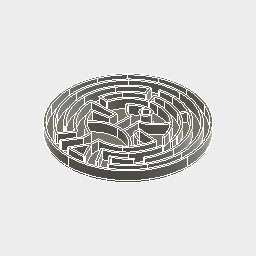
Maze (Autodesk Fusion 360 design; units mm, degrees)
Autodesk Fusion 360 part; units mm, degrees
sketch "Sketch5" plane through (0, 0, 0) normal (0, 1, 0) x (1, 0, 0)
  spline S0 degree 3 poles (-3.4402, 73.5513) (-20.4265, 73.5513) (-36.3809, 66.9367) (-48.3929, 54.9246) knots 0 0 0 0 1 1 1 1
  spline S1 degree 3 poles (-48.3929, 54.9246) (-60.405, 42.9125) (-66.9932, 26.9846) (-66.9932, 9.9983) knots 0 0 0 0 1 1 1 1
  spline S2 degree 3 poles (-66.9932, 9.9983) (-66.9932, -1.3523) (-63.9504, -12.4912) (-58.2354, -22.2279) knots 0 0 0 0 1 1 1 1
  spline S3 degree 3 poles (-58.2354, -22.2279) (-52.6792, -31.6735) (-44.7152, -39.5581) (-35.2167, -45.0615) knots 0 0 0 0 1 1 1 1
  spline S4 degree 3 poles (-35.2167, -45.0615) (-34.7404, -45.326) (-34.1319, -45.1937) (-33.8144, -44.7439) knots 0 0 0 0 1 1 1 1
  line L0 (-33.8144, -44.7439) -> (-23.9984, -30.8269)
  spline S5 degree 3 poles (-23.9984, -30.8269) (-23.6544, -30.3506) (-23.7867, -29.6892) (-24.2629, -29.3452) knots 0 0 0 0 1 1 1 1
  spline S6 degree 3 poles (-24.2629, -29.3452) (-24.2894, -29.3188) (-24.3423, -29.3188) (-24.3688, -29.2923) knots 0 0 0 0 1 1 1 1
  spline S7 degree 3 poles (-24.3688, -29.2923) (-37.8096, -21.8575) (-46.5673, -6.9085) (-46.8848, 8.9665) knots 0 0 0 0 1 1 1 1
  line L1 (-46.8848, 8.9665) -> (-20.9027, 9.9454)
  line L2 (-20.9027, 9.9454) -> (-20.9027, 4.786)
  line L3 (-20.9027, 4.786) -> (-38.1271, 1.7963)
  spline S8 degree 3 poles (-38.1271, 1.7963) (-38.7356, 1.6904) (-39.1325, 1.0554) (-38.9738, 0.4733) knots 0 0 0 0 1 1 1 1
  spline S9 degree 3 poles (-38.9738, 0.4733) (-35.8782, -11.1154) (-27.3586, -20.4023) (-16.1402, -24.5298) knots 0 0 0 0 1 1 1 1
  line L4 (-16.1402, -24.5298) -> (-16.1402, -32.8377)
  line L5 (-16.1402, -32.8377) -> (-25.7711, -48.1835)
  spline S10 degree 3 poles (-25.7711, -48.1835) (-26.0886, -48.6863) (-25.9298, -49.3213) (-25.4271, -49.6388) knots 0 0 0 0 1 1 1 1
  spline S11 degree 3 poles (-25.4271, -49.6388) (-25.2419, -49.7446) (-25.0567, -49.7975) (-24.8715, -49.7975) knots 0 0 0 0 1 1 1 1
  spline S12 degree 3 poles (-24.8715, -49.7975) (-24.5275, -49.7975) (-24.1836, -49.6123) (-23.9719, -49.2948) knots 0 0 0 0 1 1 1 1
  line L6 (-23.9719, -49.2948) -> (-14.0236, -33.4198)
  line L7 (-14.0236, -33.4198) -> (-14.0236, -23.7625)
  spline S13 degree 3 poles (-14.0236, -23.7625) (-14.0236, -23.3127) (-14.3146, -22.9158) (-14.738, -22.7571) knots 0 0 0 0 1 1 1 1
  spline S14 degree 3 poles (-14.738, -22.7571) (-19.7915, -21.0108) (-24.263, -18.1798) (-27.9407, -14.5285) knots 0 0 0 0 1 1 1 1
  spline S15 degree 3 poles (-27.9407, -14.5285) (-22.0934, -6.935) (-12.9917, -2.4106) (-3.4403, -2.4106) knots 0 0 0 0 1 1 1 1
  spline S16 degree 3 poles (-3.4403, -2.4106) (6.8785, -2.4106) (15.5568, -6.6704) (21.1131, -14.4756) knots 0 0 0 0 1 1 1 1
  spline S17 degree 3 poles (21.1131, -14.4756) (20.0018, -15.825) (18.8377, -16.9627) (17.6735, -17.8888) knots 0 0 0 0 1 1 1 1
  spline S18 degree 3 poles (17.6735, -17.8888) (12.0379, -22.3867) (4.9471, -24.6621) (-3.4402, -24.6621) knots 0 0 0 0 1 1 1 1
  spline S19 degree 3 poles (-3.4402, -24.6621) (-4.0223, -24.6621) (-4.4986, -25.1383) (-4.4986, -25.7204) knots 0 0 0 0 1 1 1 1
  line L8 (-4.4986, -25.7204) -> (-4.4986, -34.4517)
  line L9 (-4.4986, -34.4517) -> (-13.6267, -51.0675)
  spline S20 degree 3 poles (-13.6267, -51.0675) (-13.8119, -51.385) (-13.8119, -51.7819) (-13.6002, -52.1258) knots 0 0 0 0 1 1 1 1
  spline S21 degree 3 poles (-13.6002, -52.1258) (-13.415, -52.4433) (-13.0711, -52.655) (-12.7006, -52.655) knots 0 0 0 0 1 1 1 1
  line L10 (-12.7006, -52.655) -> (5.291, -52.655)
  spline S22 degree 3 poles (5.291, -52.655) (5.6614, -52.655) (6.0054, -52.4698) (6.1906, -52.1523) knots 0 0 0 0 1 1 1 1
  spline S23 degree 3 poles (6.1906, -52.1523) (6.3758, -51.8348) (6.4023, -51.4379) (6.2171, -51.1204) knots 0 0 0 0 1 1 1 1
  line L11 (6.2171, -51.1204) -> (-2.3819, -34.4517)
  line L12 (-2.3819, -34.4517) -> (-2.3819, -26.7523)
  spline S24 degree 3 poles (-2.3819, -26.7523) (6.0318, -26.5671) (13.2021, -24.1594) (18.9964, -19.5556) knots 0 0 0 0 1 1 1 1
  spline S25 degree 3 poles (18.9964, -19.5556) (25.0289, -14.7667) (30.6381, -4.5008) (33.3104, 6.5852) knots 0 0 0 0 1 1 1 1
  spline S26 degree 3 poles (33.3104, 6.5852) (33.3898, 6.8762) (33.3104, 7.1937) (33.1516, 7.4319) knots 0 0 0 0 1 1 1 1
  spline S27 degree 3 poles (33.1516, 7.4319) (32.9664, 7.67) (32.7018, 7.8552) (32.4108, 7.8817) knots 0 0 0 0 1 1 1 1
  line L13 (32.4108, 7.8817) -> (10.9796, 10.2629)
  spline S28 degree 3 poles (10.9796, 10.2629) (10.6885, 10.2894) (10.371, 10.21) (10.1594, 9.9983) knots 0 0 0 0 1 1 1 1
  spline S29 degree 3 poles (10.1594, 9.9983) (9.9477, 9.7867) (9.8154, 9.5221) (9.8154, 9.2046) knots 0 0 0 0 1 1 1 1
  line L14 (9.8154, 9.2046) -> (9.8154, 2.8546)
  spline S30 degree 3 poles (9.8154, 2.8546) (9.8154, 2.4577) (10.0535, 2.0608) (10.4239, 1.9021) knots 0 0 0 0 1 1 1 1
  line L15 (10.4239, 1.9021) -> (20.531, -2.8604)
  spline S31 degree 3 poles (20.531, -2.8604) (21.0602, -3.0985) (21.6952, -2.8869) (21.9333, -2.3577) knots 0 0 0 0 1 1 1 1
  spline S32 degree 3 poles (21.9333, -2.3577) (22.1714, -1.8285) (21.9598, -1.1935) (21.4306, -0.9554) knots 0 0 0 0 1 1 1 1
  line L16 (21.4306, -0.9554) -> (11.9056, 3.516)
  line L17 (11.9056, 3.516) -> (11.9056, 8.014)
  line L18 (11.9056, 8.014) -> (30.9556, 5.8973)
  spline S33 degree 3 poles (30.9556, 5.8973) (29.1035, -1.2465) (26.0079, -7.914) (22.4625, -12.7558) knots 0 0 0 0 1 1 1 1
  spline S34 degree 3 poles (22.4625, -12.7558) (17.7529, -6.4323) (11.0854, -2.3577) (3.1744, -0.9025) knots 0 0 0 0 1 1 1 1
  line L19 (3.1744, -0.9025) -> (3.1744, 16.269)
  spline S35 degree 3 poles (3.1744, 16.269) (11.6146, 18.174) (18.4937, 26.6671) (23.1504, 33.4669) knots 0 0 0 0 1 1 1 1
  spline S36 degree 3 poles (23.1504, 33.4669) (25.6639, 30.6887) (27.6748, 27.4873) (29.0506, 23.9154) knots 0 0 0 0 1 1 1 1
  spline S37 degree 3 poles (29.0506, 23.9154) (30.4529, 20.3171) (30.4529, 20.3171) (31.1937, 16.5071) knots 0 0 0 0 1 1 1 1
  line L20 (31.1937, 16.5071) -> (31.2202, 16.4012)
  spline S38 degree 3 poles (31.2202, 16.4012) (31.326, 15.8985) (31.7493, 15.5546) (32.2521, 15.5546) knots 0 0 0 0 1 1 1 1
  spline S39 degree 3 poles (32.2521, 15.5546) (32.3314, 15.5546) (32.3843, 15.5546) (32.4637, 15.581) knots 0 0 0 0 1 1 1 1
  spline S40 degree 3 poles (32.4637, 15.581) (33.0458, 15.6869) (33.4162, 16.2425) (33.2839, 16.8246) knots 0 0 0 0 1 1 1 1
  line L21 (33.2839, 16.8246) -> (33.2575, 16.9304)
  spline S41 degree 3 poles (33.2575, 16.9304) (32.4637, 20.8727) (32.4373, 20.9521) (31.0085, 24.6827) knots 0 0 0 0 1 1 1 1
  spline S42 degree 3 poles (31.0085, 24.6827) (25.8227, 38.0971) (12.3025, 46.7754) (-3.4402, 46.7754) knots 0 0 0 0 1 1 1 1
  spline S43 degree 3 poles (-3.4402, 46.7754) (-6.3771, 46.7754) (-9.2346, 46.4315) (-11.9863, 45.77) knots 0 0 0 0 1 1 1 1
  line L22 (-11.9863, 45.77) -> (-13.7854, 52.1729)
  spline S44 degree 3 poles (-13.7854, 52.1729) (-10.3723, 53.0196) (-6.8533, 53.4429) (-3.3079, 53.4429) knots 0 0 0 0 1 1 1 1
  spline S45 degree 3 poles (-3.3079, 53.4429) (3.386, 53.4429) (9.7889, 52.0406) (15.7156, 49.3154) knots 0 0 0 0 1 1 1 1
  spline S46 degree 3 poles (15.7156, 49.3154) (26.2725, 44.4206) (34.1306, 35.8217) (37.8877, 25.0531) knots 0 0 0 0 1 1 1 1
  spline S47 degree 3 poles (37.8877, 25.0531) (38.311, 23.836) (38.6021, 23.0423) (38.8137, 22.4602) knots 0 0 0 0 1 1 1 1
  spline S48 degree 3 poles (38.8137, 22.4602) (39.3958, 20.8992) (39.4752, 20.714) (40.2425, 16.9304) knots 0 0 0 0 1 1 1 1
  spline S49 degree 3 poles (40.2425, 16.9304) (40.3483, 16.4277) (40.7717, 16.0838) (41.2744, 16.0838) knots 0 0 0 0 1 1 1 1
  spline S50 degree 3 poles (41.2744, 16.0838) (41.3537, 16.0838) (41.4067, 16.0838) (41.486, 16.1102) knots 0 0 0 0 1 1 1 1
  spline S51 degree 3 poles (41.486, 16.1102) (42.0681, 16.2161) (42.4385, 16.7717) (42.3062, 17.3538) knots 0 0 0 0 1 1 1 1
  spline S52 degree 3 poles (42.3062, 17.3538) (41.5125, 21.2961) (41.4066, 21.5871) (40.7981, 23.2275) knots 0 0 0 0 1 1 1 1
  spline S53 degree 3 poles (40.7981, 23.2275) (40.56, 23.8361) (40.2954, 24.5769) (39.8721, 25.7675) knots 0 0 0 0 1 1 1 1
  spline S54 degree 3 poles (39.8721, 25.7675) (36.2208, 36.2979) (28.786, 44.8704) (18.8377, 50.1621) knots 0 0 0 0 1 1 1 1
  line L23 (18.8377, 50.1621) -> (21.6423, 56.1681)
  spline S55 degree 3 poles (21.6423, 56.1681) (38.6021, 46.9342) (49.0796, 29.3659) (49.0796, 10.0248) knots 0 0 0 0 1 1 1 1
  spline S56 degree 3 poles (49.0796, 10.0248) (49.0796, 0.7115) (46.6189, -8.4166) (41.9358, -16.4071) knots 0 0 0 0 1 1 1 1
  spline S57 degree 3 poles (41.9358, -16.4071) (41.6448, -16.9098) (41.8035, -17.5712) (42.3062, -17.8623) knots 0 0 0 0 1 1 1 1
  spline S58 degree 3 poles (42.3062, -17.8623) (42.465, -17.9681) (42.6502, -17.9946) (42.8354, -17.9946) knots 0 0 0 0 1 1 1 1
  spline S59 degree 3 poles (42.8354, -17.9946) (43.2058, -17.9946) (43.5498, -17.8094) (43.7614, -17.4654) knots 0 0 0 0 1 1 1 1
  spline S60 degree 3 poles (43.7614, -17.4654) (48.6033, -9.1575) (51.1698, 0.3675) (51.1698, 10.0513) knots 0 0 0 0 1 1 1 1
  spline S61 degree 3 poles (51.1698, 10.0513) (51.1698, 30.5565) (39.8456, 49.1567) (21.6158, 58.6023) knots 0 0 0 0 1 1 1 1
  spline S62 degree 3 poles (21.6158, 58.6023) (13.9164, 62.5975) (5.2381, 64.6877) (-3.4667, 64.6877) knots 0 0 0 0 1 1 1 1
  spline S63 degree 3 poles (-3.4667, 64.6877) (-8.2556, 64.6877) (-13.0181, 64.0527) (-17.6219, 62.8356) knots 0 0 0 0 1 1 1 1
  spline S64 degree 3 poles (-17.6219, 62.8356) (-18.1775, 62.6769) (-18.5215, 62.0948) (-18.3627, 61.5392) knots 0 0 0 0 1 1 1 1
  spline S65 degree 3 poles (-18.3627, 61.5392) (-18.204, 60.9836) (-17.6219, 60.6396) (-17.0663, 60.7984) knots 0 0 0 0 1 1 1 1
  spline S66 degree 3 poles (-17.0663, 60.7984) (-12.6477, 61.989) (-8.0704, 62.5711) (-3.4667, 62.5711) knots 0 0 0 0 1 1 1 1
  spline S67 degree 3 poles (-3.4667, 62.5711) (4.6825, 62.5711) (12.4877, 60.7454) (19.7373, 57.1736) knots 0 0 0 0 1 1 1 1
  line L24 (19.7373, 57.1736) -> (16.9327, 51.0881)
  spline S68 degree 3 poles (16.9327, 51.0881) (16.8268, 51.141) (16.721, 51.194) (16.5887, 51.2469) knots 0 0 0 0 1 1 1 1
  spline S69 degree 3 poles (16.5887, 51.2469) (10.3975, 54.1308) (3.6771, 55.586) (-3.3344, 55.586) knots 0 0 0 0 1 1 1 1
  spline S70 degree 3 poles (-3.3344, 55.586) (-7.4354, 55.586) (-11.4836, 55.0569) (-15.3994, 53.9721) knots 0 0 0 0 1 1 1 1
  spline S71 degree 3 poles (-15.3994, 53.9721) (-15.955, 53.8133) (-16.299, 53.2312) (-16.1402, 52.6756) knots 0 0 0 0 1 1 1 1
  spline S72 degree 3 poles (-16.1402, 52.6756) (-16.1402, 52.6492) (-16.1402, 52.6492) (-16.1138, 52.6227) knots 0 0 0 0 1 1 1 1
  spline S73 degree 3 poles (-16.1138, 52.6227) (-16.1138, 52.5962) (-16.1138, 52.5962) (-16.1138, 52.5698) knots 0 0 0 0 1 1 1 1
  line L25 (-16.1138, 52.5698) -> (-14.05, 45.2144)
  spline S74 degree 3 poles (-14.05, 45.2144) (-25.7446, 41.6954) (-35.2167, 32.4614) (-38.7621, 20.3435) knots 0 0 0 0 1 1 1 1
  line L26 (-38.7621, 20.3435) -> (-45.5619, 20.714)
  spline S75 degree 3 poles (-45.5619, 20.714) (-44.0538, 26.6406) (-41.2492, 32.2762) (-37.4127, 37.0652) knots 0 0 0 0 1 1 1 1
  spline S76 degree 3 poles (-37.4127, 37.0652) (-33.3646, 42.1187) (-28.1523, 46.2992) (-22.3315, 49.1302) knots 0 0 0 0 1 1 1 1
  spline S77 degree 3 poles (-22.3315, 49.1302) (-21.8288, 49.3683) (-21.5906, 49.9504) (-21.8023, 50.4531) knots 0 0 0 0 1 1 1 1
  line L27 (-21.8023, 50.4531) -> (-25.1096, 58.9463)
  spline S78 degree 3 poles (-25.1096, 58.9463) (-25.2155, 59.2108) (-25.4271, 59.4225) (-25.6917, 59.5548) knots 0 0 0 0 1 1 1 1
  spline S79 degree 3 poles (-25.6917, 59.5548) (-25.9563, 59.6606) (-26.2738, 59.6606) (-26.5384, 59.5283) knots 0 0 0 0 1 1 1 1
  spline S80 degree 3 poles (-26.5384, 59.5283) (-35.8252, 55.1892) (-43.6834, 48.3365) (-49.2925, 39.711) knots 0 0 0 0 1 1 1 1
  spline S81 degree 3 poles (-49.2925, 39.711) (-55.034, 30.874) (-58.0767, 20.5817) (-58.0767, 9.9983) knots 0 0 0 0 1 1 1 1
  spline S82 degree 3 poles (-58.0767, 9.9983) (-58.0767, -6.1942) (-50.9594, -21.4342) (-38.5505, -31.8588) knots 0 0 0 0 1 1 1 1
  spline S83 degree 3 poles (-38.5505, -31.8588) (-38.3652, -32.0175) (-38.1007, -32.0969) (-37.8625, -32.0969) knots 0 0 0 0 1 1 1 1
  spline S84 degree 3 poles (-37.8625, -32.0969) (-37.5715, -32.0969) (-37.254, -31.9646) (-37.0423, -31.7265) knots 0 0 0 0 1 1 1 1
  spline S85 degree 3 poles (-37.0423, -31.7265) (-36.6719, -31.2767) (-36.7248, -30.6152) (-37.1746, -30.2448) knots 0 0 0 0 1 1 1 1
  spline S86 degree 3 poles (-37.1746, -30.2448) (-49.1073, -20.2171) (-55.9336, -5.5592) (-55.9336, 9.9983) knots 0 0 0 0 1 1 1 1
  spline S87 degree 3 poles (-55.9336, 9.9983) (-55.9336, 20.1848) (-53.0232, 30.0537) (-47.4934, 38.5733) knots 0 0 0 0 1 1 1 1
  spline S88 degree 3 poles (-47.4934, 38.5733) (-42.3075, 46.5373) (-35.1109, 52.9402) (-26.6442, 57.1206) knots 0 0 0 0 1 1 1 1
  line L28 (-26.6442, 57.1206) -> (-24.0777, 50.5854)
  spline S89 degree 3 poles (-24.0777, 50.5854) (-29.8192, 47.6485) (-34.9786, 43.4417) (-39.0002, 38.3881) knots 0 0 0 0 1 1 1 1
  spline S90 degree 3 poles (-39.0002, 38.3881) (-43.2865, 33.0171) (-46.3557, 26.6406) (-47.8638, 19.9467) knots 0 0 0 0 1 1 1 1
  spline S91 degree 3 poles (-47.8638, 19.9467) (-47.8638, 19.8937) (-47.8902, 19.8408) (-47.8902, 19.7614) knots 0 0 0 0 1 1 1 1
  spline S92 degree 3 poles (-47.8902, 19.7614) (-47.9167, 19.1794) (-47.4669, 18.6767) (-46.8848, 18.6502) knots 0 0 0 0 1 1 1 1
  line L29 (-46.8848, 18.6502) -> (-37.9684, 18.1739)
  spline S93 degree 3 poles (-37.9684, 18.1739) (-37.598, 18.1475) (-37.254, 18.3327) (-37.0423, 18.6502) knots 0 0 0 0 1 1 1 1
  spline S94 degree 3 poles (-37.0423, 18.6502) (-36.963, 18.756) (-36.91, 18.8619) (-36.8836, 18.9942) knots 0 0 0 0 1 1 1 1
  spline S95 degree 3 poles (-36.8836, 18.9942) (-33.6821, 30.9798) (-24.3688, 40.0814) (-12.833, 43.3358) knots 0 0 0 0 1 1 1 1
  spline S96 degree 3 poles (-12.833, 43.3358) (-12.78, 43.3358) (-12.7271, 43.3094) (-12.6742, 43.3094) knots 0 0 0 0 1 1 1 1
  spline S97 degree 3 poles (-12.6742, 43.3094) (-12.5684, 43.3094) (-12.489, 43.3094) (-12.3832, 43.3623) knots 0 0 0 0 1 1 1 1
  spline S98 degree 3 poles (-12.3832, 43.3623) (-12.2244, 43.4152) (-12.1186, 43.4681) (-11.9863, 43.5739) knots 0 0 0 0 1 1 1 1
  spline S99 degree 3 poles (-11.9863, 43.5739) (-9.2346, 44.2883) (-6.3507, 44.6587) (-3.3873, 44.6587) knots 0 0 0 0 1 1 1 1
  spline S100 degree 3 poles (-3.3873, 44.6587) (6.4552, 44.6587) (15.3716, 41.0869) (21.6952, 35.0014) knots 0 0 0 0 1 1 1 1
  spline S101 degree 3 poles (21.6952, 35.0014) (17.0914, 28.2281) (10.1858, 19.5498) (1.9837, 18.1739) knots 0 0 0 0 1 1 1 1
  spline S102 degree 3 poles (1.9837, 18.1739) (1.481, 18.0946) (1.1106, 17.6448) (1.1106, 17.1421) knots 0 0 0 0 1 1 1 1
  line L30 (1.1106, 17.1421) -> (1.1106, -0.585)
  spline S103 degree 3 poles (1.1106, -0.585) (-0.3446, -0.3998) (-1.8528, -0.3204) (-3.3873, -0.3204) knots 0 0 0 0 1 1 1 1
  spline S104 degree 3 poles (-3.3873, -0.3204) (-4.8161, -0.3204) (-6.2184, -0.4263) (-7.6207, -0.6115) knots 0 0 0 0 1 1 1 1
  line L31 (-7.6207, -0.6115) -> (-7.6207, 17.0892)
  spline S105 degree 3 poles (-7.6207, 17.0892) (-7.5942, 17.5919) (-7.9382, 18.0681) (-8.4409, 18.1739) knots 0 0 0 0 1 1 1 1
  spline S106 degree 3 poles (-8.4409, 18.1739) (-13.6796, 19.3117) (-17.913, 22.5396) (-21.379, 28.0165) knots 0 0 0 0 1 1 1 1
  spline S107 degree 3 poles (-21.379, 28.0165) (-17.8071, 31.5619) (-13.3886, 33.9431) (-8.5467, 34.9221) knots 0 0 0 0 1 1 1 1
  spline S108 degree 3 poles (-8.5467, 34.9221) (-9.2875, 33.8902) (-9.7373, 32.6467) (-9.7373, 31.2708) knots 0 0 0 0 1 1 1 1
  spline S109 degree 3 poles (-9.7373, 31.2708) (-9.7373, 27.8312) (-6.9592, 25.0531) (-3.5196, 25.0531) knots 0 0 0 0 1 1 1 1
  spline S110 degree 3 poles (-3.5196, 25.0531) (-0.0801, 25.0531) (2.6981, 27.8312) (2.6981, 31.2708) knots 0 0 0 0 1 1 1 1
  spline S111 degree 3 poles (2.6981, 31.2708) (2.6981, 34.6575) (-0.0271, 37.4092) (-3.3873, 37.4885) knots 0 0 0 0 1 1 1 1
  line L32 (-3.3873, 37.4885) -> (-3.3873, 37.5679)
  spline S112 degree 3 poles (-3.3873, 37.5679) (-11.0338, 37.5679) (-18.1511, 34.4987) (-23.4163, 28.969) knots 0 0 0 0 1 1 1 1
  spline S113 degree 3 poles (-23.4163, 28.969) (-23.4428, 28.9425) (-23.4428, 28.9425) (-23.4692, 28.916) knots 0 0 0 0 1 1 1 1
  spline S114 degree 3 poles (-23.4692, 28.916) (-23.7867, 28.5721) (-23.8661, 28.0694) (-23.6015, 27.646) knots 0 0 0 0 1 1 1 1
  spline S115 degree 3 poles (-23.6015, 27.646) (-19.9238, 21.5342) (-15.373, 17.83) (-9.7109, 16.3483) knots 0 0 0 0 1 1 1 1
  line L33 (-9.7109, 16.3483) -> (-9.7109, -0.9554)
  spline S116 degree 3 poles (-9.7109, -0.9554) (-17.3838, -2.49) (-24.3953, -6.7233) (-29.3165, -12.994) knots 0 0 0 0 1 1 1 1
  spline S117 degree 3 poles (-29.3165, -12.994) (-32.5709, -9.3162) (-35.058, -4.9242) (-36.5132, -0.0823) knots 0 0 0 0 1 1 1 1
  line L34 (-36.5132, -0.0823) -> (-18.6803, 3.0398)
  line L35 (-18.6803, 3.0398) -> (-18.6803, 12.1679)
  line L36 (-18.6803, 12.1679) -> (-47.9432, 11.0567)
  spline S118 degree 3 poles (-47.9432, 11.0567) (-48.5252, 11.0302) (-48.975, 10.554) (-48.9486, 9.9719) knots 0 0 0 0 1 1 1 1
  spline S119 degree 3 poles (-48.9486, 9.9719) (-48.9486, 9.9454) (-48.9486, 9.919) (-48.9486, 9.8925) knots 0 0 0 0 1 1 1 1
  line L37 (-48.9486, 9.8925) -> (-49.0279, 9.8925)
  spline S120 degree 3 poles (-49.0279, 9.8925) (-49.0279, -6.6704) (-40.1909, -22.4131) (-26.4061, -30.5358) knots 0 0 0 0 1 1 1 1
  line L38 (-26.4061, -30.5358) -> (-35.005, -42.7067)
  spline S121 degree 3 poles (-35.005, -42.7067) (-43.8156, -37.415) (-51.1975, -29.9802) (-56.4098, -21.1167) knots 0 0 0 0 1 1 1 1
  spline S122 degree 3 poles (-56.4098, -21.1167) (-61.9396, -11.724) (-64.8765, -0.929) (-64.8765, 10.0513) knots 0 0 0 0 1 1 1 1
  spline S123 degree 3 poles (-64.8765, 10.0513) (-64.8765, 26.4554) (-58.4736, 41.9071) (-46.8848, 53.4958) knots 0 0 0 0 1 1 1 1
  spline S124 degree 3 poles (-46.8848, 53.4958) (-35.2961, 65.0846) (-19.8444, 71.4875) (-3.4402, 71.4875) knots 0 0 0 0 1 1 1 1
  spline S125 degree 3 poles (-3.4402, 71.4875) (12.9639, 71.4875) (28.4156, 65.0846) (40.0044, 53.4958) knots 0 0 0 0 1 1 1 1
  spline S126 degree 3 poles (40.0044, 53.4958) (51.5931, 41.9071) (57.996, 26.4554) (57.996, 10.0513) knots 0 0 0 0 1 1 1 1
  spline S127 degree 3 poles (57.996, 10.0513) (57.996, -0.929) (55.0592, -11.6975) (49.5294, -21.1167) knots 0 0 0 0 1 1 1 1
  spline S128 degree 3 poles (49.5294, -21.1167) (44.2906, -30.0067) (36.8823, -37.4415) (28.0452, -42.7331) knots 0 0 0 0 1 1 1 1
  line L39 (28.0452, -42.7331) -> (22.78, -36.5419)
  spline S129 degree 3 poles (22.78, -36.5419) (28.0981, -33.4727) (34.5539, -29.6627) (38.3904, -25.0854) knots 0 0 0 0 1 1 1 1
  spline S130 degree 3 poles (38.3904, -25.0854) (38.7608, -24.6356) (38.7079, -23.9742) (38.2581, -23.6037) knots 0 0 0 0 1 1 1 1
  spline S131 degree 3 poles (38.2581, -23.6037) (37.8083, -23.2333) (37.1468, -23.2862) (36.7764, -23.736) knots 0 0 0 0 1 1 1 1
  spline S132 degree 3 poles (36.7764, -23.736) (33.0458, -28.181) (26.4841, -31.9646) (21.2454, -35.0073) knots 0 0 0 0 1 1 1 1
  line L40 (21.2454, -35.0073) -> (20.6369, -35.3512)
  spline S133 degree 3 poles (20.6369, -35.3512) (20.3723, -35.51) (20.1871, -35.7746) (20.1341, -36.0921) knots 0 0 0 0 1 1 1 1
  spline S134 degree 3 poles (20.1341, -36.0921) (20.0812, -36.4096) (20.1606, -36.7271) (20.3723, -36.9652) knots 0 0 0 0 1 1 1 1
  line L41 (20.3723, -36.9652) -> (27.0133, -44.7969)
  spline S135 degree 3 poles (27.0133, -44.7969) (27.225, -45.035) (27.516, -45.1673) (27.8335, -45.1673) knots 0 0 0 0 1 1 1 1
  spline S136 degree 3 poles (27.8335, -45.1673) (28.0187, -45.1673) (28.2039, -45.1144) (28.3627, -45.035) knots 0 0 0 0 1 1 1 1
  spline S137 degree 3 poles (28.3627, -45.035) (37.8612, -39.5581) (45.7987, -31.6471) (51.3814, -22.2014) knots 0 0 0 0 1 1 1 1
  spline S138 degree 3 poles (51.3814, -22.2014) (57.1229, -12.4648) (60.1391, -1.3258) (60.1391, 10.0248) knots 0 0 0 0 1 1 1 1
  spline S139 degree 3 poles (60.1391, 10.0248) (60.1391, 27.0111) (53.5245, 42.9654) (41.5125, 54.9775) knots 0 0 0 0 1 1 1 1
  spline S140 degree 3 poles (41.5125, 54.9775) (29.5004, 66.9631) (13.546, 73.5513) (-3.4402, 73.5513) knots 0 0 0 0 1 1 1 1
  line L42 (-10.9279, -50.5119) -> (-3.4667, -36.9652)
  line L43 (-3.4667, -36.9652) -> (3.5712, -50.5119)
  line L44 (3.5712, -50.5119) -> (-10.9279, -50.5119)
  spline S141 degree 3 poles (0.5285, 31.2973) (0.5285, 29.0483) (-1.3236, 27.1963) (-3.5725, 27.1963) knots 0 0 0 0 1 1 1 1
  spline S142 degree 3 poles (-3.5725, 27.1963) (-5.8215, 27.1963) (-7.6736, 29.0483) (-7.6736, 31.2973) knots 0 0 0 0 1 1 1 1
  spline S143 degree 3 poles (-7.6736, 31.2973) (-7.6736, 33.5463) (-5.8215, 35.3983) (-3.5725, 35.3983) knots 0 0 0 0 1 1 1 1
  spline S144 degree 3 poles (-3.5725, 35.3983) (-1.3236, 35.3983) (0.5285, 33.5463) (0.5285, 31.2973) knots 0 0 0 0 1 1 1 1
  spline S145 degree 3 poles (9.7889, -33.9225) (16.8268, -31.8058) (23.3885, -27.7842) (28.8125, -22.2544) knots 0 0 0 0 1 1 1 1
  spline S146 degree 3 poles (28.8125, -22.2544) (35.5064, -15.4281) (40.5071, -2.9133) (42.3062, 5.8179) knots 0 0 0 0 1 1 1 1
  spline S147 degree 3 poles (42.3062, 5.8179) (42.4121, 6.4) (42.0681, 6.9556) (41.486, 7.0614) knots 0 0 0 0 1 1 1 1
  spline S148 degree 3 poles (41.486, 7.0614) (40.9039, 7.1673) (40.3483, 6.8233) (40.2425, 6.2412) knots 0 0 0 0 1 1 1 1
  spline S149 degree 3 poles (40.2425, 6.2412) (37.7554, -5.7973) (31.8023, -16.2219) (27.3308, -20.7727) knots 0 0 0 0 1 1 1 1
  spline S150 degree 3 poles (27.3308, -20.7727) (21.8275, -26.3819) (15.1071, -30.3506) (7.9104, -32.2821) knots 0 0 0 0 1 1 1 1
  spline S151 degree 3 poles (7.9104, -32.2821) (7.3548, -32.4408) (7.0108, -33.0229) (7.1696, -33.5785) knots 0 0 0 0 1 1 1 1
  spline S152 degree 3 poles (7.1696, -33.5785) (7.1696, -33.605) (7.1696, -33.605) (7.196, -33.6315) knots 0 0 0 0 1 1 1 1
  spline S153 degree 3 poles (7.196, -33.6315) (7.2225, -33.7638) (7.2754, -33.8696) (7.3283, -33.9754) knots 0 0 0 0 1 1 1 1
  line L45 (7.3283, -33.9754) -> (17.1179, -49.3213)
  spline S154 degree 3 poles (17.1179, -49.3213) (17.3296, -49.6388) (17.6735, -49.7975) (18.0175, -49.7975) knots 0 0 0 0 1 1 1 1
  spline S155 degree 3 poles (18.0175, -49.7975) (18.2027, -49.7975) (18.4144, -49.7446) (18.5731, -49.6388) knots 0 0 0 0 1 1 1 1
  spline S156 degree 3 poles (18.5731, -49.6388) (19.0758, -49.3213) (19.2081, -48.6598) (18.8906, -48.1835) knots 0 0 0 0 1 1 1 1
  line L46 (18.8906, -48.1835) -> (9.7889, -33.9225)
  spline S157 degree 3 poles (-3.7048, 81.4358) (-43.1542, 81.4358) (-75.1423, 49.4477) (-75.1423, 9.9983) knots 0 0 0 0 1 1 1 1
  spline S158 degree 3 poles (-75.1423, 9.9983) (-75.1423, -29.451) (-43.1542, -61.4392) (-3.7048, -61.4392) knots 0 0 0 0 1 1 1 1
  spline S159 degree 3 poles (-3.7048, -61.4392) (35.7446, -61.4392) (67.7327, -29.451) (67.7327, 9.9983) knots 0 0 0 0 1 1 1 1
  spline S160 degree 3 poles (67.7327, 9.9983) (67.7327, 49.4477) (35.7446, 81.4358) (-3.7048, 81.4358) knots 0 0 0 0 1 1 1 1
  spline S161 degree 3 poles (45.3225, -39.029) (38.946, -45.4054) (31.5377, -50.406) (23.2827, -53.8985) knots 0 0 0 0 1 1 1 1
  spline S162 degree 3 poles (23.2827, -53.8985) (14.7366, -57.5233) (5.6614, -59.349) (-3.7048, -59.349) knots 0 0 0 0 1 1 1 1
  spline S163 degree 3 poles (-3.7048, -59.349) (-13.0711, -59.349) (-22.1463, -57.5233) (-30.6923, -53.8985) knots 0 0 0 0 1 1 1 1
  spline S164 degree 3 poles (-30.6923, -53.8985) (-38.9473, -50.406) (-46.3557, -45.4054) (-52.7321, -39.029) knots 0 0 0 0 1 1 1 1
  spline S165 degree 3 poles (-52.7321, -39.029) (-59.1086, -32.6525) (-64.1092, -25.2442) (-67.6017, -16.9892) knots 0 0 0 0 1 1 1 1
  spline S166 degree 3 poles (-67.6017, -16.9892) (-71.2265, -8.4431) (-73.0521, 0.6321) (-73.0521, 9.9983) knots 0 0 0 0 1 1 1 1
  spline S167 degree 3 poles (-73.0521, 9.9983) (-73.0521, 19.3646) (-71.2265, 28.4398) (-67.6017, 36.9858) knots 0 0 0 0 1 1 1 1
  spline S168 degree 3 poles (-67.6017, 36.9858) (-64.1092, 45.2408) (-59.1086, 52.6492) (-52.7321, 59.0256) knots 0 0 0 0 1 1 1 1
  spline S169 degree 3 poles (-52.7321, 59.0256) (-46.3556, 65.4021) (-38.9473, 70.4027) (-30.6923, 73.8952) knots 0 0 0 0 1 1 1 1
  spline S170 degree 3 poles (-30.6923, 73.8952) (-22.1463, 77.52) (-13.0711, 79.3456) (-3.7048, 79.3456) knots 0 0 0 0 1 1 1 1
  spline S171 degree 3 poles (-3.7048, 79.3456) (5.6614, 79.3456) (14.7366, 77.52) (23.2827, 73.8952) knots 0 0 0 0 1 1 1 1
  spline S172 degree 3 poles (23.2827, 73.8952) (31.5377, 70.4027) (38.946, 65.4021) (45.3225, 59.0256) knots 0 0 0 0 1 1 1 1
  spline S173 degree 3 poles (45.3225, 59.0256) (51.6989, 52.6492) (56.6996, 45.2408) (60.1921, 36.9858) knots 0 0 0 0 1 1 1 1
  spline S174 degree 3 poles (60.1921, 36.9858) (63.8169, 28.4398) (65.6425, 19.3646) (65.6425, 9.9983) knots 0 0 0 0 1 1 1 1
  spline S175 degree 3 poles (65.6425, 9.9983) (65.6425, 0.6321) (63.8168, -8.4431) (60.1921, -16.9892) knots 0 0 0 0 1 1 1 1
  spline S176 degree 3 poles (60.1921, -16.9892) (56.6731, -25.2442) (51.6725, -32.6525) (45.3225, -39.029) knots 0 0 0 0 1 1 1 1
extrude "Extrude2" add sketch "Sketch5" along normal blind 10 makes body 1 at (-46.3185, 0, 34.8138) makes body 2 at (37.9945, 4.4444, 7.5802) makes body 3 at (-7.3346, 3.3333, -81.3452)
sketch "Sketch6" plane through (0, 0, 0) normal (0, 1, 0) x (1, 0, 0)
  circle A0 centre (-3.7048, 9.9983) radius 71.4375
  constraint coincident A0 origin
  constraint coincident A0
extrude "Extrude3" add sketch "Sketch6" against normal blind 2 bodies 1 2 3
